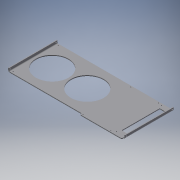
# Autodesk Inventor part: Plate
Saved by Autodesk Inventor 2018 (Build 220112000, 112)
## iProperties
Created: 2020-03-13
Part Number: Plate
Material: Generic
Document SubType Name: Sheet Metal
Designer: tomah
Density: 1 g/cm^3
Sheet Metal Rule: Default
Appearance: Default
Author: tomah
Autodesk Inventor part; units mm, degrees
ref_plane "YZ Plane" through (0, 0, 0) normal (1, 0, 0) x (0, 1, 0)
ref_plane "XZ Plane" through (0, 0, 0) normal (0, 1, 0) x (-1, 0, 0)
ref_plane "XY Plane" through (0, 0, 0) normal (0, 0, 1) x (1, 0, 0)
sketch "Sketch1" plane through (0, 0, 0) normal (0, 1, 0) x (-1, 0, 0)
  line L0 (0, 0) -> (-428.625, 0)
  line L1 (-428.625, 0) -> (-428.625, 177.8)
  line L2 (-428.625, 177.8) -> (0, 177.8)
  line L3 (0, 177.8) -> (0, 0)
  dimension "d0" = 428.625
  dimension "d1" = 177.8
  measures "d0" distance of L0.start L0.end
  measures "d1" distance of L0.end L1.end
extrude "Plate1" add sketch "Sketch1" along normal blind 3.048
sketch "Sketch2" plane through (3.048, 0, 177.8) normal (-1, 0, 0) x (0, -1, 0)
  line L0 (0, -177.8) -> (0, 0)
  line L1 (0, 0) -> (-12.7, 0)
  line L2 (-12.7, 0) -> (-12.7, -177.8)
  line L3 (-12.7, -177.8) -> (0, -177.8)
  constraints: 6 end point, 1 horizontal, 1 perpendicular, 1 vertical
edge flange "Flange1" height 12.7 angle 90 thickness 3.048 bend radius 3.048 thickness toward (-1, 0, 0) relief tear relief width 3.048 relief depth 1.524 corner gap 3.048 corner form 0 edges at (0, 3.048, 88.9) (428.625, 3.048, 88.9) wall of the first edge with corners at (3.048, 0, 0) (3.048, 0, 177.8) (3.048, 12.7, 177.8) (3.048, 12.7, 0)
bend "Bend1"
corner "Corner1"
sketch "Sketch3" plane through (0, 12.7, 0) normal (-1, 0, 0) x (0, 0, 1)
  line L0 (0, -6.604) -> (0, 0) projected
  line L1 (0, 0) -> (177.8, 0) projected
  line L2 (177.8, -12.7) -> (0, -12.7) projected
  line L3 (177.8, 0) -> (177.8, -6.604) projected
  line L4 (4.7625, -4.445) -> (173.0375, -4.445) construction
  line L5 (88.9, 0) -> (88.9, -12.7) construction
  dimension "d13" = 168.275
  dimension "d14" = 4.445
  constraints: 4 end point, 2 midpoint, 1 horizontal, 1 symmetric about line
  measures "d13" distance of L4.start L4.end
  measures "d14" distance from line of L1 L4.start
hole "Hole1" at (0, 8.255, 4.7625) at (0, 8.255, 173.0375) direction (1, 0, 0) diameter 4 end through all
sketch "Sketch4" plane through (0, 0, 0) normal (0, -1, 0) x (1, 0, 0)
  line L0 (428.625, 177.8) -> (428.625, 0) projected
  line L1 (0, 0) -> (0, 177.8) projected
  line L2 (422.529, 177.8) -> (6.096, 177.8) projected
  line L3 (6.096, 0) -> (422.529, 0) projected
  line L4 (422.529, 0) -> (422.529, 177.8) projected
  line L5 (396.875, 158.75) -> (415.925, 158.75)
  line L6 (415.925, 158.75) -> (415.925, 19.05)
  line L7 (415.925, 19.05) -> (396.875, 19.05)
  line L8 (396.875, 19.05) -> (396.875, 158.75)
  dimension "d22" = 31.75
  dimension "d23" = 19.05
  dimension "d24" = 19.05
  dimension "d25" = 19.05
  constraints: 8 end point, 2 parallel, 1 horizontal, 1 perpendicular
  measures "d22" distance between parallel lines of L0 L8
  measures "d23" distance of L5.start L5.end
  measures "d24" distance between parallel lines of L2 L5
  measures "d25" distance between parallel lines of L3 L7
extrude "Cut1" cut sketch "Sketch4" against normal blind 3.048
sketch "Sketch5" plane through (0, 0, 0) normal (0, -1, 0) x (1, 0, 0)
  line L0 (422.529, 177.8) -> (6.096, 177.8) projected
  line L1 (6.096, 177.8) -> (6.096, 0) construction
  line L2 (6.096, 0) -> (422.529, 0) projected
  line L3 (422.529, 0) -> (422.529, 177.8) projected
  line L4 (12.446, 171.45) -> (390.525, 171.45) construction
  line L5 (390.525, 171.45) -> (390.525, 6.35) construction
  line L6 (390.525, 6.35) -> (12.446, 6.35) construction
  line L7 (12.446, 6.35) -> (12.446, 171.45) construction
  line L8 (396.875, 19.05) -> (396.875, 158.75) projected
  point P0 (0, 0)
  dimension "d28" = 6.35
  dimension "d29" = 6.35
  dimension "d30" = 6.35
  dimension "d31" = 6.35
  constraints: 8 end point, 4 coincident, 2 parallel, 1 horizontal, 1 perpendicular
  measures "d28" distance between parallel lines of L1 L7
  measures "d29" distance between parallel lines of L0 L4
  measures "d30" distance between parallel lines of L2 L6
  measures "d31" distance between parallel lines of L8 L5
hole "Hole2" at (12.446, 0, 171.45) at (12.446, 0, 6.35) at (390.525, 0, 6.35) at (390.525, 0, 171.45) direction (0, 1, 0) diameter 3 end through all
sketch "Sketch6" plane through (0, 0, 0) normal (0, -1, 0) x (1, 0, 0)
  line L0 (422.529, 177.8) -> (6.096, 177.8) projected
  line L1 (6.096, 177.8) -> (6.096, 0) projected
  line L2 (422.529, 0) -> (422.529, 177.8) projected
  line L3 (6.096, 0) -> (422.529, 0) projected
  circle A0 centre (72.7, 88.9) radius 60
  circle A1 centre (201.2875, 88.9) radius 60
  circle A2 centre (329.875, 88.9) radius 60
  line L4 (72.7, 88.9) -> (329.875, 88.9) construction
  line L5 (12.7, 177.8) -> (12.7, 0) construction
  line L6 (0, 0) -> (0, 177.8) projected
  dimension "d39" = 120
  dimension "d40" = 120
  dimension "d41" = 120
  dimension "d42" = 257.175
  dimension "d43" = 128.5875
  dimension "d44" = 177.8
  dimension "d45" = 88.9
  dimension "d46" = 12.7
  constraints: 4 end point, 3 centre point, 2 point on line, 1 horizontal, 1 midpoint, 1 tangent, 1 vertical
  measures "d39" diameter of A0
  measures "d40" diameter of A1
  measures "d41" diameter of A2
  measures "d42" distance of L4.start L4.end
  measures "d43" distance of L4.start A1.centre
  measures "d44" distance of L2.start L0.start
  measures "d45" distance between parallel lines of L3 L4
  measures "d46" distance between parallel lines of L6 L5
extrude "Cut2" cut sketch "Sketch6" against normal blind 3.048 contours A0 | A1
sketch "Sketch8" plane through (0, 0, 0) normal (0, -1, 0) x (1, 0, 0)
  line L0 (422.529, 177.8) -> (6.096, 177.8)
  line L1 (422.529, 177.8) -> (6.096, 177.8)
  line L2 (270.129, 177.8) -> (422.529, 177.8)
  line L3 (422.529, 177.8) -> (422.529, 184.15)
  line L4 (422.529, 184.15) -> (270.129, 184.15)
  line L5 (270.129, 184.15) -> (270.129, 177.8)
  point P0 (0, 0)
  dimension "d55" = 6.35
  dimension "d56" = 152.4
  measures "d55" distance of L2.end L3.end
  measures "d56" distance of L3.end L4.end
sheet face with bend "Face2" sketch "Sketch8" thickness 3.048 toward (0, 1, 0) bend radius 3.048 relief tear relief width 3.048 relief depth 1.524
bend "Bend2"
sketch "Sketch7" plane through (0, 0, 0) normal (0, -1, 0) x (1, 0, 0)
  line L0 (422.529, 177.8) -> (6.096, 177.8) construction
  line L1 (6.096, 0) -> (422.529, 0) construction
  line L2 (396.875, 19.05) -> (396.875, 158.75) construction
  line L3 (276.225, 179.375) -> (377.825, 179.375) construction
  line L4 (377.825, 179.375) -> (377.825, 4.775) construction
  line L5 (377.825, 4.775) -> (276.225, 4.775) construction
  line L6 (276.225, 4.775) -> (276.225, 179.375) construction
  line L7 (276.225, 92.075) -> (377.825, 92.075) construction
  point P0 (0, 0)
  dimension "d49" = 101.6
  dimension "d50" = 174.6
  dimension "d51" = 177.8
  dimension "d52" = 85.725
  dimension "d53" = 19.05
  constraints: 10 end point, 4 coincident, 2 midpoint, 2 parallel, 1 horizontal, 1 perpendicular
  measures "d49" distance of L3.start L3.end
  measures "d50" distance of L5.end L3.start
  measures "d51" distance between parallel lines of L1 L0
  measures "d52" distance between parallel lines of L0 L7
  measures "d53" distance between parallel lines of L2 L4
hole "Hole3" at (276.225, 0, 179.375) at (377.825, 0, 179.375) at (377.825, 0, 4.775) at (276.225, 0, 4.775) at (276.225, 0, 179.375) direction (0, 1, 0) diameter 3 end through all
fillet "Corner Round1" radius 3.175 3 edges at (270.129, 1.524, 184.15) (270.129, 1.524, 177.8) (422.529, 1.524, 184.15)
equation "\"d20\" = Thickness"
equation "\"d25\" = d24"
equation "\"d26\" = Thickness"
equation "\"d29\" = d28"
equation "\"d30\" = d28"
equation "\"d31\" = d28"
equation "\"d37\" = Thickness"
equation "\"d43\" = 0.5 * d42"
equation "\"d45\" = 0.5 * d44"
equation "\"d47\" = Thickness"
equation "\"d67\" = Thickness"
equation "\"d2\" = Thickness"
equation "\"d3\" = BendReliefWidth"
equation "\"d4\" = BendReliefDepth"
equation "\"d5\" = MinimumRemnant"
equation "\"d6\" = TransitionRadius"
equation "\"d9\" = BendRadius"
equation "\"d10\" = CornerReliefSize"
equation "\"d11\" = GapSize"
equation "\"d12\" = JacobiRadiusSize"
equation "\"d57\" = BendRadius"
equation "\"d58\" = BendReliefWidth"
equation "\"d60\" = MinimumRemnant"
equation "\"d59\" = BendReliefDepth"
equation "\"d61\" = TransitionRadius"
equation "\"BendRadius\" = Thickness"
equation "\"BendReliefWidth\" = Thickness"
equation "\"BendReliefDepth\" = 0.5 * Thickness"
equation "\"CornerReliefSize\" = 4 * Thickness"
equation "\"MinimumRemnant\" = 2 * Thickness"
equation "\"TransitionRadius\" = BendRadius"
equation "\"JacobiRadiusSize\" = Thickness"
equation "\"GapSize\" = Thickness"
equation "\"Thickness\" = 3.048"
body "Solid1"
